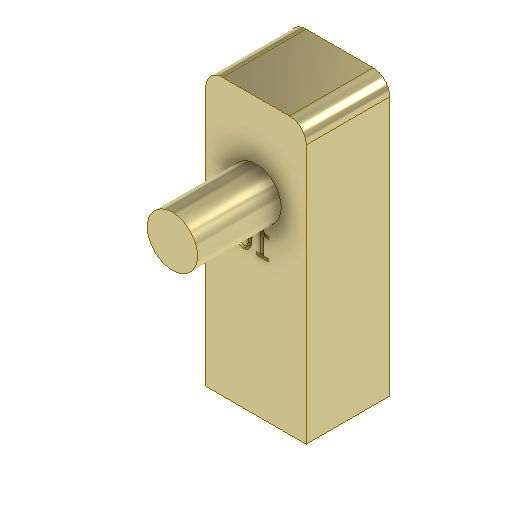
# Autodesk Inventor part: fengmingplayerleg
Saved by Autodesk Inventor 2025 (Build 290162000, 162)
## iProperties
Created: 2024-11-17
Part Number: fengmingplayerleg
Material: Generic
Document SubType Name: Modeling
Designer: wj
Density: 1 g/cm^3
Appearance: Gold - Metal
Author: wj
Autodesk Inventor part; units mm, degrees
ref_plane "YZ Plane" through (0, 0, 0) normal (1, 0, 0) x (0, 1, 0)
ref_plane "XZ Plane" through (0, 0, 0) normal (0, 1, 0) x (-1, 0, 0)
ref_plane "XY Plane" through (0, 0, 0) normal (0, 0, 1) x (1, 0, 0)
sketch "Sketch1" plane through (0, 0, 0) normal (0, 1, 0) x (-1, 0, 0)
  line L0 (0.8095, 4.9498) -> (-11.1905, 4.9498)
  line L1 (-11.1905, 4.9498) -> (-11.1905, -5.0502)
  line L2 (-11.1905, -5.0502) -> (0.8095, -5.0502)
  line L3 (0.8095, -5.0502) -> (0.8095, 4.9498)
  point P0 (0, 0)
  dimension "d0" = 10
  dimension "d1" = 12
  constraints: 8 end point, 2 parallel, 1 horizontal, 1 perpendicular
  measures "d0" distance of L0.end L1.end
  measures "d1" distance of L1.end L2.end
extrude "Extrusion1" add sketch "Sketch1" along normal blind 33
fillet "Fillet1" radius 2 1 edges at (11.1905, 33, -0.0502)
fillet "Fillet2" radius 2 1 edges at (-0.8095, 33, -0.0502)
sketch "Sketch2" plane through (-0.8095, 0, 4.9498) normal (0, 0, 1) x (1, 0, 0)
  circle A0 centre (6, 23.0256) radius 3
  line L0 (0, 0) -> (0, 31) projected
  point P0 (0.8095, 0)
  dimension "d6" = 6
  dimension "d7" = 6
  constraints: 1 centre point
  measures "d6" diameter of A0
  measures "d7" distance from line of A0.centre L0
extrude "Extrusion2" add sketch "Sketch2" along normal blind 20
sketch "Sketch3" plane through (5.1905, 23.0256, 24.9498) normal (0, 0, 1) x (1, 0, 0)
  circle A0 centre (0, 0) radius 3
  point P0 (-5.1905, -23.0256)
  constraints: 1 centre point
extrude "Extrusion3" cut sketch "Sketch3" against normal blind 10
sketch "Sketch4" plane through (11.1905, 0, -5.0502) normal (0, 0, -1) x (-1, 0, 0)
  line L0 (10.9572, 30.4948) -> (1.3526, 30.4948)
  line L1 (1.3526, 30.4948) -> (1.3526, 3.7115)
  line L2 (1.3526, 3.7115) -> (10.9572, 3.7115)
  line L3 (10.9572, 3.7115) -> (10.9572, 30.4948)
  line L4 (4.0281, 19.7513) -> (8.6026, 19.7513) construction
  line L5 (8.6026, 19.7513) -> (8.6026, 16.5774) construction
  line L6 (8.6026, 16.5774) -> (4.0281, 16.5774) construction
  line L7 (4.0281, 16.5774) -> (4.0281, 19.7513) construction
  line L8 (5.977, 16.6416) -> (4.49, 16.6416)
  line L9 (4.49, 16.6416) -> (4.49, 16.9528)
  line L10 (4.49, 16.9528) -> (5.0433, 16.9528)
  line L11 (5.0433, 16.9528) -> (5.0433, 18.9955)
  line L12 (5.0433, 18.9955) -> (4.49, 18.9955)
  line L13 (4.49, 18.9955) -> (4.49, 19.2746)
  spline S0 degree 2 poles (4.49, 19.2746) (4.8037, 19.2746) (5.1001, 19.4524) (5.1199, 19.6995) knots 0 0 0 1 2 2 2
  line L14 (5.1199, 19.6995) -> (5.4361, 19.6995)
  line L15 (5.4361, 19.6995) -> (5.4361, 16.9528)
  line L16 (5.4361, 16.9528) -> (5.977, 16.9528)
  line L17 (5.977, 16.9528) -> (5.977, 16.6416)
  spline S1 degree 2 poles (8.4347, 18.1656) (8.4347, 17.3455) (7.9579, 16.5774) (7.4615, 16.5774) knots 0 0 0 1 2 2 2
  spline S2 degree 2 poles (7.4615, 16.5774) (6.9576, 16.5774) (6.4858, 17.3603) (6.4858, 18.1631) knots 0 0 0 1 2 2 2
  spline S3 degree 2 poles (6.4858, 18.1631) (6.4858, 18.9881) (6.9625, 19.7513) (7.4615, 19.7513) knots 0 0 0 1 2 2 2
  spline S4 degree 2 poles (7.4615, 19.7513) (7.9629, 19.7513) (8.4347, 18.9609) (8.4347, 18.1656) knots 0 0 0 1 2 2 2
  spline S5 degree 2 poles (7.911, 17.2368) (7.9703, 17.3875) (8.0197, 17.8519) (8.0197, 18.1656) knots 0 0 0 1 2 2 2
  spline S6 degree 2 poles (8.0197, 18.1656) (8.0197, 18.4793) (7.9703, 18.9412) (7.9085, 19.0968) knots 0 0 0 1 2 2 2
  spline S7 degree 2 poles (7.9085, 19.0968) (7.8468, 19.2524) (7.6319, 19.4129) (7.4615, 19.4129) knots 0 0 0 1 2 2 2
  spline S8 degree 2 poles (7.4615, 19.4129) (7.291, 19.4129) (7.0712, 19.2524) (7.007, 19.0918) knots 0 0 0 1 2 2 2
  spline S9 degree 2 poles (7.007, 19.0918) (6.9452, 18.9362) (6.9008, 18.462) (6.9008, 18.1631) knots 0 0 0 1 2 2 2
  spline S10 degree 2 poles (6.9008, 18.1631) (6.9008, 17.842) (6.9403, 17.4122) (7.0045, 17.2443) knots 0 0 0 1 2 2 2
  spline S11 degree 2 poles (7.0045, 17.2443) (7.0638, 17.0862) (7.2836, 16.9157) (7.4615, 16.9157) knots 0 0 0 1 2 2 2
  spline S12 degree 2 poles (7.4615, 16.9157) (7.6294, 16.9157) (7.8493, 17.0763) (7.911, 17.2368) knots 0 0 0 1 2 2 2
  point P0 (11.1905, 0)
  constraints: 8 end point, 2 parallel, 1 horizontal, 1 perpendicular, 2 other
extrude "Extrusion4" cut sketch "Sketch4" against normal blind 20 contours L8 L9 L10 L11 L12 L13 S0 L14 L15 L16 L17 | S1 S2 S3 S4
body "Solid1"
